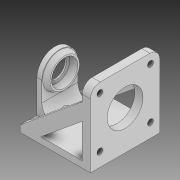
# Autodesk Inventor part: Winder_driver
Saved by Autodesk Inventor 2020 (Build 240168000, 168)
## iProperties
Created: 2021-03-13
Part Number: Winder_driver
Material: Generic
Document SubType Name: Modeling
Designer: DDeGo
Density: 1 g/cm^3
Appearance: Default
Author: DDeGo
Autodesk Inventor part; units mm, degrees
ref_plane "YZ Plane" through (0, 0, 0) normal (1, 0, 0) x (0, 1, 0)
ref_plane "XZ Plane" through (0, 0, 0) normal (0, 1, 0) x (-1, 0, 0)
ref_plane "XY Plane" through (0, 0, 0) normal (0, 0, 1) x (1, 0, 0)
sketch "Sketch3" plane through (0, 0, 0) normal (0, 0, 1) x (1, 0, 0)
  line L0 (0, 0) -> (0, 35)
  line L1 (0, 35) -> (3, 35)
  line L2 (3, 35) -> (3, 4)
  line L3 (3, 4) -> (38, 4)
  line L4 (38, 4) -> (38, 0)
  line L5 (38, 0) -> (0, 0)
  line L6 (0, 25) -> (3, 25) construction
  dimension "d0" = 10
  dimension "d1" = 25
  dimension "d2" = 35
  dimension "d3" = 4
  dimension "d4" = 3
  constraints: 14 end point, 5 perpendicular, 2 point on line, 1 horizontal, 1 vertical
  measures "d0" distance between parallel lines of L1 L6
  measures "d1" distance between parallel lines of L5 L6
  measures "d2" distance of L2.end L3.end
  measures "d3" distance between parallel lines of L5 L3
  measures "d4" distance of L0.end L1.end
extrude "Extrusion1" add sketch "Sketch3" along normal mid plane 22
sketch "Sketch4" plane through (3, 4, -11) normal (1, 0, 0) x (0, 0, -1)
  line L0 (0, 31) -> (-22, 31) construction
  line L1 (-11, 31) -> (-11, 20) construction
  circle A0 centre (-11, 20) radius 8.05
  point P0 (-11, -4)
  dimension "d7" = 11
  dimension "d8" = 16.1
  constraints: 2 end point, 1 centre point, 1 coincident, 1 midpoint, 1 vertical
  measures "d7" distance of L1.start L1.end
  measures "d8" diameter of A0
extrude "Extrusion2" cut sketch "Sketch4" against normal through all
fillet "Fillet3" radius 8 1 edges at (3, 4, 0)
sketch "Sketch5" plane through (3, 4, -11) normal (0, 1, 0) x (1, 0, 0)
  line L0 (35, 0) -> (35, -22) construction
  line L1 (35, -11) -> (0, -11) construction
  line L2 (0, 0) -> (0, -22) construction
  circle A0 centre (7, -11) radius 2.6
  circle A1 centre (28, -11) radius 2.6
  point P0 (-3, -11)
  dimension "d11" = 7
  dimension "d12" = 7
  dimension "d13" = 5.2
  constraints: 2 centre point, 2 end point, 2 midpoint, 2 point on line, 1 equal radius
  measures "d11" distance from line of L0 A1.centre
  measures "d12" distance from line of L2 A0.centre
  measures "d13" diameter of A0
extrude "Extrusion3" cut sketch "Sketch5" along normal mid plane 24.75
sketch "Sketch6" plane through (0, 0, 0) normal (0, 0, 1) x (1, 0, 0)
  line L0 (3, 15.95) -> (0, 15.95) construction
  line L1 (0, 15.95) -> (0, 17.95)
  line L2 (0, 17.95) -> (1, 17.95)
  line L3 (1, 17.95) -> (1, 15.95)
  line L4 (0, 15.95) -> (0, 32.05) construction
  line L5 (1, 15.95) -> (0, 15.95)
  line L6 (3, 32.05) -> (3, 15.95) construction
  line L7 (3, 15.95) -> (6, 15.95)
  line L8 (6, 15.95) -> (6, 14.95)
  line L9 (6, 14.95) -> (3, 13.45)
  line L10 (3, 13.45) -> (3, 15.95)
  line L11 (0, 24) -> (3, 24) construction
  point P0 (0, 0)
  dimension "d16" = 1
  dimension "d17" = 2
  dimension "d18" = 5
  dimension "d19" = 2.5
  dimension "d20" = 1
  constraints: 18 end point, 5 perpendicular, 2 midpoint, 1 horizontal, 1 point on line, 1 vertical
  measures "d16" distance between parallel lines of L1 L3
  measures "d17" distance of L2.end L3.end
  measures "d18" distance between parallel lines of L8 L3
  measures "d19" distance of L9.end L0.start
  measures "d20" distance of L7.end L8.end
revolve "Revolution1" add sketch "Sketch6" angle 360 about axis through (0, 24, 0) along (1, 0, 0)
fillet "Fillet1" radius 11 2 edges at (1.5, 35, 11) (1.5, 35, -11)
sketch "Sketch7" plane through (38, 0, 11) normal (1, 0, 0) x (0, 0, -1)
  circle A0 centre (11, 24) radius 6.05 construction
  line L0 (-10.25, 2.75) -> (32.25, 2.75) construction
  line L1 (32.25, 2.75) -> (32.25, 45.25)
  line L2 (32.25, 45.25) -> (-10.25, 45.25)
  line L3 (-10.25, 45.25) -> (-10.25, 2.75)
  line L4 (-10.25, 2.75) -> (32.25, 45.25) construction
  line L5 (32.25, 2.75) -> (-10.25, 45.25) construction
  line L6 (-10.25, 2.75) -> (-10.25, 0)
  line L7 (-10.25, 0) -> (32.25, 0)
  line L8 (32.25, 0) -> (32.25, 2.75)
  line L9 (22, 0) -> (0, 0) projected
  circle A1 centre (11, 24) radius 11
  line L10 (26.5, 8.5) -> (-4.5, 8.5) construction
  line L11 (-4.5, 8.5) -> (-4.5, 39.5) construction
  line L12 (-4.5, 39.5) -> (26.5, 39.5) construction
  line L13 (26.5, 39.5) -> (26.5, 8.5) construction
  line L14 (26.5, 8.5) -> (-4.5, 39.5) construction
  line L15 (-4.5, 8.5) -> (26.5, 39.5) construction
  circle A2 centre (-4.5, 39.5) radius 1.75
  circle A3 centre (-4.5, 8.5) radius 1.75
  circle A4 centre (26.5, 8.5) radius 1.75
  circle A5 centre (26.5, 39.5) radius 1.75
  point P0 (11, 0)
  point P1 (11, 0)
  dimension "d23" = 42.5
  dimension "d24" = 22
  dimension "d25" = 31
  dimension "d26" = 3.5
  constraints: 30 end point, 6 midpoint, 5 centre point, 5 coincident, 5 perpendicular, 4 parallel, 3 equal radius, 2 horizontal, 1 point on line, 1 vertical
  measures "d23" distance of L1.end L2.end
  measures "d24" diameter of A1
  measures "d25" distance of L11.end L12.end
  measures "d26" diameter of A2
extrude "Extrusion4" add sketch "Sketch7" along normal blind 5
sketch "Sketch8" plane through (38, 0, 11) normal (-1, 0, 0) x (0, 0, 1)
  line L0 (10.25, 0) -> (0, 0)
  line L1 (0, 0) -> (0, 4)
  line L2 (0, 4) -> (10.25, 4)
  line L3 (10.25, 4) -> (10.25, 0)
  line L4 (-22, 4) -> (-22, 0) projected
  line L5 (-32.25, 0) -> (-32.25, 45.25) projected
  line L6 (-22, 4) -> (-32.25, 4)
  line L7 (-32.25, 4) -> (-32.25, 0)
  line L8 (-32.25, 0) -> (-22, 0)
  line L9 (-22, 0) -> (-22, 4)
  point P0 (-11, 0)
  constraints: 16 end point, 4 parallel, 2 horizontal, 2 perpendicular
extrude "Extrusion5" add sketch "Sketch8" along normal up to surface (38 mm away)
sketch "Sketch9" plane through (38, 4, -21.25) normal (0, 0, -1) x (-1, 0, 0)
  line L0 (0, 9) -> (0, 31) projected
  line L1 (0, 20.8923) -> (25.405, 0)
  line L2 (0, 0) -> (38, 0) projected
  line L3 (38, 0) -> (0, 31.25)
  line L4 (0, 0) -> (0, 41.25) projected
  point P0 (38, -4)
  point P1 (0, 28)
  dimension "d31" = 8
  dimension "d40" = 10
  constraints: 4 end point, 3 point on line, 1 parallel
  measures "d31" distance between parallel lines of L1 L3
  measures "d40" distance of L4.end L3.end
extrude "Extrusion6" add sketch "Sketch9" against normal blind 3 contours L0 L4 L3 L2 L1
fillet "Fillet2" radius 4 2 edges at (38, 30.0711, -18.25) (6.2975, 4, -18.25)
mirror "Mirror1" about plane through (0, 0, 0) normal (0, 0, 1) of "Extrusion6", "Fillet2"
sketch "Sketch10" plane through (0, 4, -11) normal (0, 1, 0) x (1, 0, 0)
  circle A0 centre (10, -11) radius 2.6 projected
  circle A1 centre (10, -11) radius 4.5
  point P0 (0, -11)
  dimension "d37" = 9
  constraints: 1 centre point, 1 coincident
  measures "d37" diameter of A1
extrude "Extrusion7" cut sketch "Sketch10" along normal blind 7 contours A0 | A1
fillet "Fillet4" radius 6 2 edges at (40.5, 45.25, 21.25) (40.5, 45.25, -21.25)
body "Solid1"
